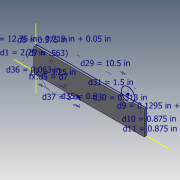
# Autodesk Inventor part: VP SWITCHMNT A
Saved by Autodesk Inventor 2018.3 (Build 223284000, 284)
## iProperties
Created: 2020-01-27
Material: Generic
Vendor: HHMI: JRC - ID&F
Document SubType Name: Modeling
Designer: arnoldj
Density: 1 g/cm^3
Appearance: Default
RuleStatus: InUse
AfterDocSave0: file://Part Number Cleaner
DESIGN DEPARTMENT: HHMI: JRC - ID&F
ALTERED ITEM PART NUMBER: N/A
ALTERED ITEM VENDOR: N/A
ALTERED ITEM DESCRIPTION: N/A
Author: arnoldj
Revision Number: 0
Autodesk Inventor part; units mm, degrees
ref_plane "YZ Plane" through (0, 0, 0) normal (1, 0, 0) x (0, 1, 0)
ref_plane "XZ Plane" through (0, 0, 0) normal (0, 1, 0) x (-1, 0, 0)
ref_plane "XY Plane" through (0, 0, 0) normal (0, 0, 1) x (1, 0, 0)
sketch "Sketch1" plane through (0, 0, 0) normal (0, 0, 1) x (1, 0, 0)
  line L0 (0, 121.6177) -> (0, -51.755) projected
  line L1 (-63.9166, 0) -> (383.4994, 0) projected
  line L2 (0, 0) -> (319.5828, 0)
  line L3 (319.5828, 0) -> (319.5828, 69.85)
  line L4 (319.5828, 69.85) -> (0, 69.85)
  line L5 (0, 69.85) -> (0, 0)
  line L6 (9.525, 14.2875) -> (92.075, 14.2875) construction
  circle A0 centre (50.8, 14.2875) radius 41.275 construction
  line L7 (0, 34.925) -> (319.5828, 34.925) construction
  circle A1 centre (266.7, 77.8002) radius 19.05
  circle A2 centre (127, 1.6002) radius 7.62
  point P0 (50.8, 55.5625)
  point P1 (310.4515, 57.15)
  point P2 (310.4515, 12.7)
  dimension "d0" = 319.5828
  dimension "d1" = 69.85
  dimension "d2" = 82.55
  dimension "d5" = 14.2875
  dimension "d7" = 14.2875
  dimension "d8" = 9.525
  dimension "d9" = 9.1313
  dimension "d10" = 22.225
  dimension "d11" = 22.225
  dimension "d29" = 266.7
  dimension "d30" = 7.9502
  dimension "d31" = 38.1
  dimension "d35" = 15.24
  dimension "d36" = 1.6002
  dimension "d37" = 127
  constraints: 12 end point, 3 centre point, 3 midpoint, 2 horizontal, 2 parallel, 2 point on circle, 2 vertical alignment, 1 coincident, 1 perpendicular
  measures "d0" distance of L3.end L4.end
  measures "d1" distance of L4.end L2.start
  measures "d2" distance of L6.start L6.end
  measures "d5" distance between parallel lines of L6 L2
  measures "d7" distance from line of A0.end L4
  measures "d8" distance from line of L0 L6.start
  measures "d9" distance from line of point (310.452, 57.15) L3
  measures "d10" distance from line of point (310.452, 57.15) L7
  measures "d11" distance from line of L7 point (310.452, 12.7)
  measures "d29" distance from line of point (266.7, 77.8) L0
  measures "d30" distance from line of point (266.7, 77.8) L4
  measures "d31" diameter of A1
  measures "d35" diameter of A2
  measures "d36" distance from line of L2 A2.centre
  measures "d37" distance from line of A2.centre L0
extrude "Extrusion1" add sketch "Sketch1" along normal blind 5.842 contours L4 A1 L3 L1 A2 L0 | L4 A1 | A2 L1 picked at (261.678, 68.614) picked at (126.7265, 4.018)
hole "Hole1" at (310.4515, 57.15, 0) at (310.4515, 12.7, 0) direction (0, 0, 1) diameter 3.81 end through all
hole "Hole2" at (9.525, 14.2875, 0) at (92.075, 14.2875, 0) at (50.8, 55.5625, 0) direction (0, 0, 1) diameter 5.588 end through all
fillet "Fillet1" radius 6.35 2 edges at (0, 69.85, 2.921) (0, 0, 2.921)
extrude "Extrusion2" cut sketch "Sketch1" along normal up to next contours A1 L4 | L4 A1 | A2 L1 | L1 A2
fillet "Fillet2" radius 3.175 4 edges at (249.3882, 69.85, 2.921) (284.0118, 69.85, 2.921) (134.4501, 0, 2.921) (119.5499, 0, 2.921)
sketch "Sketch2" plane through (0, 0, 5.842) normal (0, 0, 1) x (1, 0, 0)
  point P0 (0, 0)
equation "\"d5\" = d7"
body "Solid1"
